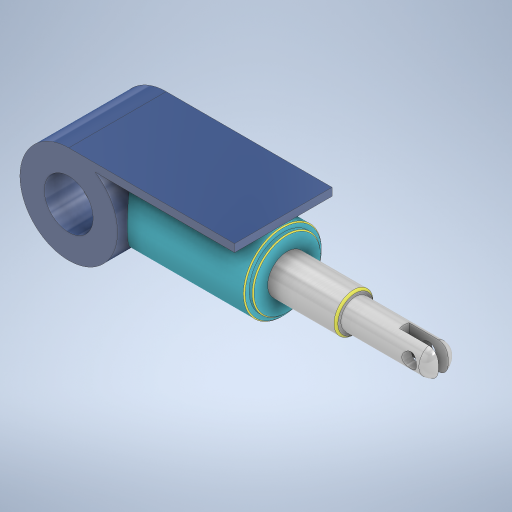
# Autodesk Inventor part: Hydraulic Arm
Saved by Autodesk Inventor 2024 (Build 280153000, 153)
## iProperties
Created: 2023-06-06
Part Number: Hydraulic Arm
Material: Generic
Document SubType Name: Modeling
Designer: vilas
Density: 1 g/cm^3
Appearance: Default
Author: vilas
Autodesk Inventor part; units mm, degrees
ref_plane "YZ Plane" through (0, 0, 0) normal (1, 0, 0) x (0, 1, 0)
ref_plane "XZ Plane" through (0, 0, 0) normal (0, 1, 0) x (-1, 0, 0)
ref_plane "XY Plane" through (0, 0, 0) normal (0, 0, 1) x (1, 0, 0)
sketch "Sketch1" plane through (0, 0, 0) normal (0, 0, 1) x (1, 0, 0)
  circle A0 centre (0, 0) radius 25
  dimension "d0" = 50
  constraints: 1 centre point, 1 coincident
  measures "d0" diameter of A0
extrude "Extrusion1" add sketch "Sketch1" along normal mid plane 50
sketch "Sketch2" plane through (0, 0, 0) normal (1, 0, 0) x (0, 1, 0)
  circle A0 centre (0, 0) radius 20
  line L0 (25, 25) -> (-25, 25) projected
  line L1 (-25, -25) -> (25, -25) projected
  line L2 (25, 25) -> (21, 25)
  line L3 (21, 25) -> (21, -25)
  line L4 (21, -25) -> (25, -25)
  line L5 (25, -25) -> (25, 25)
  dimension "d3" = 40
  dimension "d4" = 4
  constraints: 8 end point, 2 parallel, 1 centre point, 1 coincident, 1 horizontal, 1 perpendicular, 1 point on line
  measures "d3" diameter of A0
  measures "d4" distance of L4.end L3.end
extrude "Extrusion2" add sketch "Sketch2" along normal blind 85
sketch "Sketch3" plane through (0, 0, 0) normal (0, 0, 1) x (1, 0, 0)
  circle A0 centre (0, 0) radius 12.5
  dimension "d7" = 25
  constraints: 1 centre point, 1 coincident
  measures "d7" diameter of A0
extrude "Extrusion3" cut sketch "Sketch3" along normal through all both and the other way through all
sketch "Sketch4" plane through (85, 0, 0) normal (1, 0, 0) x (0, 0, -1)
  circle A0 centre (0, 0) radius 17.5
  dimension "d10" = 35
  constraints: 1 centre point, 1 coincident
  measures "d10" diameter of A0
extrude "Extrusion4" add sketch "Sketch4" along normal blind 2
sketch "Sketch5" plane through (87, 0, 0) normal (1, 0, 0) x (0, 0, -1)
  circle A0 centre (0, 0) radius 10
  dimension "d13" = 20
  constraints: 1 centre point, 1 coincident
  measures "d13" diameter of A0
extrude "Extrusion5" add sketch "Sketch5" along normal blind 35
sketch "Sketch6" plane through (122, 0, 0) normal (1, 0, 0) x (0, 0, -1)
  circle A0 centre (0, 0) radius 7.5
  dimension "d16" = 15
  constraints: 1 centre point, 1 coincident
  measures "d16" diameter of A0
extrude "Extrusion6" add sketch "Sketch6" along normal blind 45
sketch "Sketch7" plane through (0, 0, 0) normal (0, 0, 1) x (1, 0, 0)
  circle A0 centre (157, 0) radius 3.75
  line L0 (167, -7.5) -> (167, 7.5) projected
  point P0 (0, 0)
  dimension "d19" = 7.5
  dimension "d20" = 10
  constraints: 1 centre point
  measures "d19" diameter of A0
  measures "d20" distance from line of L0 A0.centre
extrude "Extrusion7" cut sketch "Sketch7" along normal through all both and the other way through all
chamfer "Chamfer1" distance 0.5 angle 45 2 edges at (85, -20, 0) (87, 0, 17.5)
chamfer "Chamfer2" distance 1 angle 45 1 edges at (122, 0, 10)
fillet "Fillet1" radius 5 1 edges at (167, 0, 7.5)
sketch "Sketch8" plane through (0, 0, 0) normal (0, 0, 1) x (1, 0, 0)
  arc A0 (-12.5, 0) -> (0, -12.5) centre (0, 0) ccw
  arc A1 (-25, 0) -> (0, -25) centre (0, 0) ccw
  line L0 (0, 0) -> (-25, 0)
  line L1 (0, 0) -> (0, -25)
  dimension "d30" = 25
  dimension "d31" = 50
  constraints: 4 end point, 4 point on circle, 2 centre point, 2 coincident, 2 midpoint, 1 horizontal, 1 vertical
  measures "d30" diameter of A0
  measures "d31" diameter of A1
extrude "Extrusion8" cut sketch "Sketch8" along normal mid plane 15 contours A0 L1 A1 L0
sketch "Sketch9" plane through (0, 0, 0) normal (0, 1, 0) x (-1, 0, 0)
  line L0 (-167, -2.5) -> (-167, 2.5) projected
  line L1 (-167, -2.5) -> (-147, -2.5)
  line L2 (-147, -2.5) -> (-147, 2.5)
  line L3 (-147, 2.5) -> (-167, 2.5)
  point P0 (0, 0)
  dimension "d34" = 20
  constraints: 6 end point, 2 perpendicular, 1 horizontal
  measures "d34" distance of L0.start L1.end
extrude "Extrusion9" cut sketch "Sketch9" along normal through all both and the other way through all
body "Solid1"
